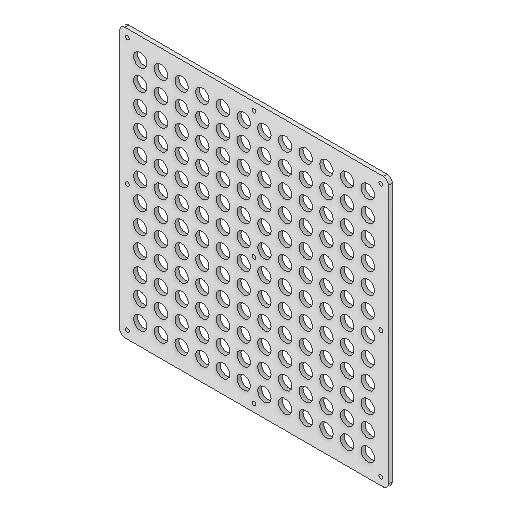
# Autodesk Inventor part: 3DP_PLA_Test_tube_array_bottom_plate
Saved by Autodesk Inventor 2025 (Build 290162010, 162A)
## iProperties
Created: 2018-06-16
Part Number: 3DP_PLA_Test_tube_array_bottom_plate
Material: ABS Plastic
Document SubType Name: Modeling
Designer: Andrzej
Density: 1.06 g/cm^3
Appearance: Smooth - White
Author: Andrzej
Autodesk Inventor part; units mm, degrees
ref_plane "YZ Plane" through (0, 0, 0) normal (1, 0, 0) x (0, 1, 0)
ref_plane "XZ Plane" through (0, 0, 0) normal (0, 1, 0) x (-1, 0, 0)
ref_plane "XY Plane" through (0, 0, 0) normal (0, 0, 1) x (1, 0, 0)
sketch "Sketch1" plane through (0, 0, 0) normal (0, 0, 1) x (1, 0, 0)
  line L0 (-114.0262, 116.9116) -> (93.9738, 116.9116)
  line L1 (93.9738, 116.9116) -> (93.9738, -91.0884)
  line L2 (93.9738, -91.0884) -> (-114.0262, -91.0884)
  line L3 (-114.0262, -91.0884) -> (-114.0262, 116.9116)
  circle A0 centre (-98.0262, 100.9116) radius 5.2
  circle A1 centre (-82.0262, 100.9116) radius 5.2
  circle A2 centre (-66.0262, 100.9116) radius 5.2
  circle A3 centre (-50.0262, 100.9116) radius 5.2
  circle A4 centre (-34.0262, 100.9116) radius 5.2
  circle A5 centre (-18.0262, 100.9116) radius 5.2
  circle A6 centre (-2.0262, 100.9116) radius 5.2
  circle A7 centre (13.9738, 100.9116) radius 5.2
  circle A8 centre (29.9738, 100.9116) radius 5.2
  circle A9 centre (45.9738, 100.9116) radius 5.2
  circle A10 centre (-98.0262, 84.9116) radius 5.2
  circle A11 centre (-82.0262, 84.9116) radius 5.2
  circle A12 centre (-66.0262, 84.9116) radius 5.2
  circle A13 centre (-50.0262, 84.9116) radius 5.2
  circle A14 centre (-34.0262, 84.9116) radius 5.2
  circle A15 centre (-18.0262, 84.9116) radius 5.2
  circle A16 centre (-2.0262, 84.9116) radius 5.2
  circle A17 centre (13.9738, 84.9116) radius 5.2
  circle A18 centre (29.9738, 84.9116) radius 5.2
  circle A19 centre (45.9738, 84.9116) radius 5.2
  circle A20 centre (-98.0262, 68.9116) radius 5.2
  circle A21 centre (-82.0262, 68.9116) radius 5.2
  circle A22 centre (-66.0262, 68.9116) radius 5.2
  circle A23 centre (-50.0262, 68.9116) radius 5.2
  circle A24 centre (-34.0262, 68.9116) radius 5.2
  circle A25 centre (-18.0262, 68.9116) radius 5.2
  circle A26 centre (-2.0262, 68.9116) radius 5.2
  circle A27 centre (13.9738, 68.9116) radius 5.2
  circle A28 centre (29.9738, 68.9116) radius 5.2
  circle A29 centre (45.9738, 68.9116) radius 5.2
  circle A30 centre (-98.0262, 52.9116) radius 5.2
  circle A31 centre (-82.0262, 52.9116) radius 5.2
  circle A32 centre (-66.0262, 52.9116) radius 5.2
  circle A33 centre (-50.0262, 52.9116) radius 5.2
  circle A34 centre (-34.0262, 52.9116) radius 5.2
  circle A35 centre (-18.0262, 52.9116) radius 5.2
  circle A36 centre (-2.0262, 52.9116) radius 5.2
  circle A37 centre (13.9738, 52.9116) radius 5.2
  circle A38 centre (29.9738, 52.9116) radius 5.2
  circle A39 centre (45.9738, 52.9116) radius 5.2
  circle A40 centre (-98.0262, 36.9116) radius 5.2
  circle A41 centre (-82.0262, 36.9116) radius 5.2
  circle A42 centre (-66.0262, 36.9116) radius 5.2
  circle A43 centre (-50.0262, 36.9116) radius 5.2
  circle A44 centre (-34.0262, 36.9116) radius 5.2
  circle A45 centre (-18.0262, 36.9116) radius 5.2
  circle A46 centre (-2.0262, 36.9116) radius 5.2
  circle A47 centre (13.9738, 36.9116) radius 5.2
  circle A48 centre (29.9738, 36.9116) radius 5.2
  circle A49 centre (45.9738, 36.9116) radius 5.2
  circle A50 centre (-98.0262, 20.9116) radius 5.2
  circle A51 centre (-82.0262, 20.9116) radius 5.2
  circle A52 centre (-66.0262, 20.9116) radius 5.2
  circle A53 centre (-50.0262, 20.9116) radius 5.2
  circle A54 centre (-34.0262, 20.9116) radius 5.2
  circle A55 centre (-18.0262, 20.9116) radius 5.2
  circle A56 centre (-2.0262, 20.9116) radius 5.2
  circle A57 centre (13.9738, 20.9116) radius 5.2
  circle A58 centre (29.9738, 20.9116) radius 5.2
  circle A59 centre (45.9738, 20.9116) radius 5.2
  circle A60 centre (-98.0262, 4.9116) radius 5.2
  circle A61 centre (-82.0262, 4.9116) radius 5.2
  circle A62 centre (-66.0262, 4.9116) radius 5.2
  circle A63 centre (-50.0262, 4.9116) radius 5.2
  circle A64 centre (-34.0262, 4.9116) radius 5.2
  circle A65 centre (-18.0262, 4.9116) radius 5.2
  circle A66 centre (-2.0262, 4.9116) radius 5.2
  circle A67 centre (13.9738, 4.9116) radius 5.2
  circle A68 centre (29.9738, 4.9116) radius 5.2
  circle A69 centre (45.9738, 4.9116) radius 5.2
  circle A70 centre (-98.0262, -11.0884) radius 5.2
  circle A71 centre (-82.0262, -11.0884) radius 5.2
  circle A72 centre (-66.0262, -11.0884) radius 5.2
  circle A73 centre (-50.0262, -11.0884) radius 5.2
  circle A74 centre (-34.0262, -11.0884) radius 5.2
  circle A75 centre (-18.0262, -11.0884) radius 5.2
  circle A76 centre (-2.0262, -11.0884) radius 5.2
  circle A77 centre (13.9738, -11.0884) radius 5.2
  circle A78 centre (29.9738, -11.0884) radius 5.2
  circle A79 centre (45.9738, -11.0884) radius 5.2
  circle A80 centre (-98.0262, -27.0884) radius 5.2
  circle A81 centre (-82.0262, -27.0884) radius 5.2
  circle A82 centre (-66.0262, -27.0884) radius 5.2
  circle A83 centre (-50.0262, -27.0884) radius 5.2
  circle A84 centre (-34.0262, -27.0884) radius 5.2
  circle A85 centre (-18.0262, -27.0884) radius 5.2
  circle A86 centre (-2.0262, -27.0884) radius 5.2
  circle A87 centre (13.9738, -27.0884) radius 5.2
  circle A88 centre (29.9738, -27.0884) radius 5.2
  circle A89 centre (45.9738, -27.0884) radius 5.2
  circle A90 centre (-98.0262, -43.0884) radius 5.2
  circle A91 centre (-82.0262, -43.0884) radius 5.2
  circle A92 centre (-66.0262, -43.0884) radius 5.2
  circle A93 centre (-50.0262, -43.0884) radius 5.2
  circle A94 centre (-34.0262, -43.0884) radius 5.2
  circle A95 centre (-18.0262, -43.0884) radius 5.2
  circle A96 centre (-2.0262, -43.0884) radius 5.2
  circle A97 centre (13.9738, -43.0884) radius 5.2
  circle A98 centre (29.9738, -43.0884) radius 5.2
  circle A99 centre (45.9738, -43.0884) radius 5.2
  circle A100 centre (61.9738, 100.9116) radius 5.2
  circle A101 centre (61.9738, 84.9116) radius 5.2
  circle A102 centre (61.9738, 68.9116) radius 5.2
  circle A103 centre (61.9738, 52.9116) radius 5.2
  circle A104 centre (61.9738, 36.9116) radius 5.2
  circle A105 centre (61.9738, 20.9116) radius 5.2
  circle A106 centre (61.9738, 4.9116) radius 5.2
  circle A107 centre (61.9738, -11.0884) radius 5.2
  circle A108 centre (61.9738, -27.0884) radius 5.2
  circle A109 centre (61.9738, -43.0884) radius 5.2
  circle A110 centre (77.9738, 100.9116) radius 5.2
  circle A111 centre (77.9738, 84.9116) radius 5.2
  circle A112 centre (77.9738, 68.9116) radius 5.2
  circle A113 centre (77.9738, 52.9116) radius 5.2
  circle A114 centre (77.9738, 36.9116) radius 5.2
  circle A115 centre (77.9738, 20.9116) radius 5.2
  circle A116 centre (77.9738, 4.9116) radius 5.2
  circle A117 centre (77.9738, -11.0884) radius 5.2
  circle A118 centre (77.9738, -27.0884) radius 5.2
  circle A119 centre (77.9738, -43.0884) radius 5.2
  circle A120 centre (-98.0262, -59.0884) radius 5.2
  circle A121 centre (-82.0262, -59.0884) radius 5.2
  circle A122 centre (-66.0262, -59.0884) radius 5.2
  circle A123 centre (-50.0262, -59.0884) radius 5.2
  circle A124 centre (-34.0262, -59.0884) radius 5.2
  circle A125 centre (-18.0262, -59.0884) radius 5.2
  circle A126 centre (-2.0262, -59.0884) radius 5.2
  circle A127 centre (13.9738, -59.0884) radius 5.2
  circle A128 centre (29.9738, -59.0884) radius 5.2
  circle A129 centre (45.9738, -59.0884) radius 5.2
  circle A130 centre (61.9738, -59.0884) radius 5.2
  circle A131 centre (77.9738, -59.0884) radius 5.2
  circle A132 centre (-98.0262, -75.0884) radius 5.2
  circle A133 centre (-82.0262, -75.0884) radius 5.2
  circle A134 centre (-66.0262, -75.0884) radius 5.2
  circle A135 centre (-50.0262, -75.0884) radius 5.2
  circle A136 centre (-34.0262, -75.0884) radius 5.2
  circle A137 centre (-18.0262, -75.0884) radius 5.2
  circle A138 centre (-2.0262, -75.0884) radius 5.2
  circle A139 centre (13.9738, -75.0884) radius 5.2
  circle A140 centre (29.9738, -75.0884) radius 5.2
  circle A141 centre (45.9738, -75.0884) radius 5.2
  circle A142 centre (61.9738, -75.0884) radius 5.2
  circle A143 centre (77.9738, -75.0884) radius 5.2
  point P0 (0, 0)
  point P1 (-108.0262, 110.9116)
  point P2 (-10.0262, 110.9116)
  point P3 (87.9738, 110.9116)
  point P4 (-108.0262, 12.9116)
  point P5 (-108.0262, -85.0884)
  point P6 (-10.0262, -85.0884)
  point P7 (87.9738, -85.0884)
  point P8 (87.9738, 12.9116)
  point P9 (-10.0262, 12.9116)
  dimension "d0" = 208
  dimension "d1" = 208
  dimension "d2" = 10.4
  dimension "d3" = 16
  dimension "d4" = 16
  dimension "d7" = 16
  dimension "d10" = 16
  dimension "d19" = 6
  dimension "d20" = 6
  dimension "d22" = 104
  dimension "d23" = 6
  dimension "d24" = 104
  dimension "d25" = 6
  constraints: 144 centre point, 8 end point, 6 horizontal alignment, 6 vertical alignment, 2 horizontal, 2 parallel, 1 perpendicular, 1 vertical, 286 other
  measures "d0" distance of L1.end L2.end
  measures "d1" distance of L0.end L1.end
  measures "d2" diameter of A0
  measures "d3" distance from line of L3 A0.centre
  measures "d4" distance from line of L0 A0.centre
  measures "d7" distance of A0.centre A1.centre
  measures "d10" distance of A0.centre A10.centre
  measures "d19" distance from line of L3 point (-108.026, 110.912)
  measures "d20" distance from line of L0 point (-108.026, 110.912)
  measures "d22" distance from line of L0 point (-108.026, 12.912)
  measures "d23" distance from line of L2 point (-108.026, -85.088)
  measures "d24" distance from line of L3 point (-10.026, 110.912)
  measures "d25" distance from line of L1 point (87.974, 110.912)
extrude "Extrusion2" add sketch "Sketch1" along normal blind 3
hole "Hole1" at (87.9738, 110.9116, 0) at (-108.0262, 12.9116, 0) at (87.9738, 12.9116, 0) at (-10.0262, 12.9116, 0) at (-10.0262, -85.0884, 0) at (-108.0262, -85.0884, 0) at (-108.0262, 110.9116, 0) at (-10.0262, 110.9116, 0) at (87.9738, -85.0884, 0) direction (0, 0, 1) diameter 3 end through all
fillet "Fillet1" radius 4 4 edges at (93.9738, 116.9116, 1.5) (93.9738, -91.0884, 1.5) (-114.0262, -91.0884, 1.5) (-114.0262, 116.9116, 1.5)
equation "\"d0\" = d1"
equation "\"d3\" = d4"
equation "\"d20\" = d19"
equation "\"d22\" = 0.5 * d1"
equation "\"d23\" = d19"
equation "\"d24\" = d22"
equation "\"d25\" = d19"
body "Solid2"
